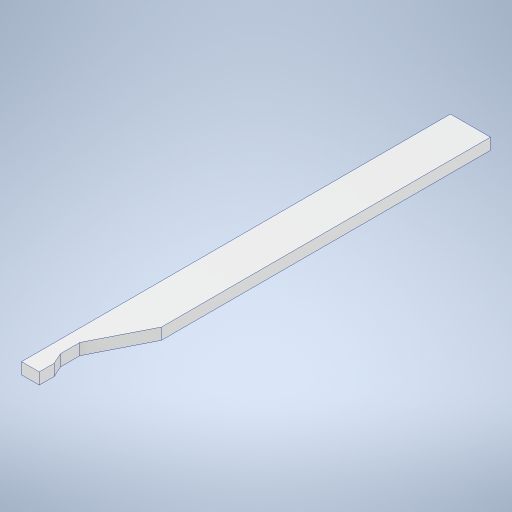
# Autodesk Inventor part: YflanecYcrepA
Saved by Autodesk Inventor 2024 (Build 280153000, 153)
## iProperties
Created: 2023-06-18
Part Number: YflanecYcrepA
Material: Aluminum 6061
Document SubType Name: Modeling
Designer: KirikDK
Density: 2.7 g/cm^3
Appearance: Aluminum - Flat
Mass: 3128.5 g
Surface Area: 1487.34 cm^2
Volume: 1158.7 cm^3
Author: KirikDK
Autodesk Inventor part; units mm, degrees
ref_plane "YZ Plane" through (0, 0, 0) normal (1, 0, 0) x (0, 1, 0)
ref_plane "XZ Plane" through (0, 0, 0) normal (0, 1, 0) x (-1, 0, 0)
ref_plane "XY Plane" through (0, 0, 0) normal (0, 0, 1) x (1, 0, 0)
sketch "Sketch1" plane through (0, 0, 0) normal (0, 1, 0) x (-1, 0, 0)
  line L0 (4, 14) -> (-86, 14)
  line L1 (-86, 14) -> (-86, -736)
  line L2 (-86, -736) -> (4, -736)
  line L3 (4, -736) -> (4, 14)
  point P0 (0, 0)
  dimension "d0" = 750
  dimension "d1" = 90
  constraints: 8 end point, 2 parallel, 1 horizontal, 1 perpendicular
  measures "d0" distance of L2.end L0.start
  measures "d1" distance of L0.start L0.end
extrude "Extrusion1" add sketch "Sketch1" along normal blind 20
sketch "Sketch2" plane through (0, 20, 0) normal (0, 1, 0) x (1, 0, 0)
  line L0 (100, -14) -> (18, -14)
  line L1 (18, -14) -> (18, 66)
  line L2 (18, 66) -> (100, 66)
  line L3 (100, 66) -> (100, -14)
  line L4 (18, 66) -> (100, 228)
  line L5 (100, 228) -> (100, 66)
  line L6 (18, 32) -> (27, 12)
  line L7 (27, 12) -> (27, -14)
  line L8 (-4, -14) -> (86, -14) projected
  point P0 (0, 0)
  dimension "d10" = 26
  dimension "d11" = 80
  dimension "d13" = 82
  dimension "d14" = 82
  dimension "d15" = 162
  dimension "d16" = 162
  dimension "d17" = 9
  dimension "d18" = 0
  dimension "d19" = 22
  dimension "d20" = 20
  constraints: 16 end point, 2 parallel, 2 perpendicular, 2 point on line, 1 horizontal, 1 vertical
  measures "d10" distance of L6.end L7.end
  measures "d11" distance of L0.end L1.end
  measures "d13" distance of L0.start L0.end
  measures "d14" distance of L1.end L2.end
  measures "d15" distance of L4.end L2.end
  measures "d16" vertical distance of L1.end L4.end
  measures "d17" horizontal distance of L6.start L6.end
  measures "d18" distance from line of L8 L0.end
  measures "d19" distance of L0.end L8.start
  measures "d20" vertical distance of L6.end L6.start
extrude "Extrusion2" cut sketch "Sketch2" against normal blind 25 contours L0 L7 L6 L1 L2 L3 | L2 L4 L5
sketch "Sketch3" plane through (0, 20, 0) normal (0, 1, 0) x (1, 0, 0)
  line L0 (86, 736) -> (-4, 736) projected
  line L1 (86, 736) -> (66, 736)
  line L2 (66, 736) -> (66, -31)
  line L3 (66, -31) -> (86, -31)
  line L4 (86, -31) -> (86, 736)
  line L5 (-4, 736) -> (-4, -14) projected
  point P0 (0, 0)
  dimension "d7" = 70
  constraints: 8 end point, 2 parallel, 1 horizontal, 1 perpendicular
  measures "d7" distance between parallel lines of L5 L2
extrude "Extrusion3" cut sketch "Sketch3" against normal blind 30
body "Solid1"
